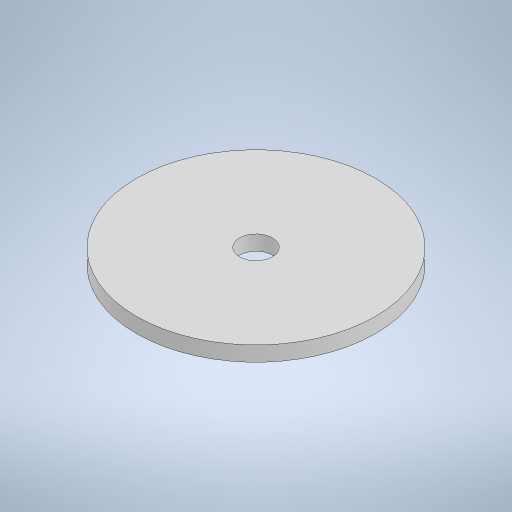
# Autodesk Inventor part: Mold Cap
Saved by Autodesk Inventor 2023.2 (Build 272271000, 271)
## iProperties
Created: 2023-06-16
Part Number: Mold Cap
Material: Generic
Document SubType Name: Modeling
Designer: Nathan Cai
Density: 1 g/cm^3
Appearance: Default
Author: Nathan Cai
Autodesk Inventor part; units mm, degrees
ref_plane "YZ Plane" through (0, 0, 0) normal (1, 0, 0) x (0, 1, 0)
ref_plane "XZ Plane" through (0, 0, 0) normal (0, 1, 0) x (-1, 0, 0)
ref_plane "XY Plane" through (0, 0, 0) normal (0, 0, 1) x (1, 0, 0)
sketch "Sketch1" plane through (0, 0, 0) normal (0, 1, 0) x (-1, 0, 0)
  circle A0 centre (0, 0) radius 1.7526
  circle A1 centre (0, 0) radius 12.7
  dimension "d0" = 3.5052
  dimension "d1" = 25.4
  constraints: 2 centre point, 2 coincident
  measures "d0" diameter of A0
  measures "d1" diameter of A1
extrude "Extrusion1" add sketch "Sketch1" along normal blind 1.5875
body "Solid1"
